Autodesk Fusion 360 part; units mm, degrees
(part 9 of 14)
  arc A2489 (70.5612, 9.5568) -> (70.5612, 10.2553) centre (70.5612, 9.906) ccw
  line L4099 (71.181, 52.94) -> (71.181, 51.54)
  arc A2490 (70.5612, 9.3472) -> (70.5612, 10.4648) centre (70.5612, 9.906) ccw
  line L4100 (83.0072, 9.779) -> (83.5152, 9.779)
  line L4101 (70.3072, 9.906) -> (70.8152, 9.906)
  arc A2491 (70.231, 9.906) -> (70.8914, 9.906) centre (70.5612, 9.906) ccw
  arc A2492 (83.5914, 9.779) -> (82.931, 9.779) centre (83.2612, 9.779) ccw
  line L4102 (70.3072, 9.906) -> (70.8152, 9.906)
  line L4103 (70.5612, 9.652) -> (70.5612, 10.16)
  arc A2493 (70.5612, 10.4648) -> (70.5612, 9.3472) centre (70.5612, 9.906) ccw
  arc A2494 (84.3788, 9.779) -> (82.1436, 9.779) centre (83.2612, 9.779) ccw
  line L4104 (70.5612, 9.652) -> (70.5612, 10.16)
  arc A2495 (71.6788, 9.906) -> (69.4436, 9.906) centre (70.5612, 9.906) ccw
  arc A2496 (83.5914, 9.779) -> (82.931, 9.779) centre (83.2612, 9.779) ccw
  line L4105 (70.3072, 9.906) -> (70.8152, 9.906)
  arc A2497 (70.5612, 10.4648) -> (70.5612, 9.3472) centre (70.5612, 9.906) ccw
  arc A2498 (70.5612, 9.3472) -> (70.5612, 10.4648) centre (70.5612, 9.906) ccw
  arc A2499 (70.231, 9.906) -> (70.8914, 9.906) centre (70.5612, 9.906) ccw
  arc A2500 (70.231, 9.906) -> (70.8914, 9.906) centre (70.5612, 9.906) ccw
  arc A2501 (70.231, 9.906) -> (70.8914, 9.906) centre (70.5612, 9.906) ccw
  line L4106 (71.181, 52.94) -> (71.181, 51.54)
  line L4107 (71.181, 52.94) -> (71.181, 51.54)
  line L4108 (70.5612, 9.652) -> (70.5612, 10.16)
  arc A2502 (72.331, 52.5562) -> (72.331, 51.9238) centre (72.331, 52.24) ccw
  line L4109 (71.181, 55.14) -> (71.181, 53.74)
  arc A2503 (70.5612, 10.4648) -> (70.5612, 9.3472) centre (70.5612, 9.906) ccw
  arc A2504 (70.8914, 9.906) -> (70.231, 9.906) centre (70.5612, 9.906) ccw
  arc A2505 (70.8914, 9.906) -> (70.231, 9.906) centre (70.5612, 9.906) ccw
  line L4110 (71.181, 55.14) -> (71.181, 53.74)
  line L4111 (69.281, 52.94) -> (69.281, 51.54)
  line L4112 (70.3072, 9.906) -> (70.8152, 9.906)
  arc A2506 (70.5612, 10.2553) -> (70.5612, 9.5568) centre (70.5612, 9.906) ccw
  line L4113 (70.3072, 9.906) -> (70.8152, 9.906)
  arc A2507 (70.231, 9.906) -> (70.8914, 9.906) centre (70.5612, 9.906) ccw
  arc A2508 (70.8914, 9.906) -> (70.231, 9.906) centre (70.5612, 9.906) ccw
  line L4114 (69.281, 55.14) -> (69.281, 53.74)
  arc A2509 (83.5914, 9.779) -> (82.931, 9.779) centre (83.2612, 9.779) ccw
  arc A2510 (70.8914, 9.906) -> (70.231, 9.906) centre (70.5612, 9.906) ccw
  line L4115 (70.5612, 9.652) -> (70.5612, 10.16)
  line L4116 (70.3072, 9.906) -> (70.8152, 9.906)
  arc A2511 (82.1436, 9.779) -> (84.3788, 9.779) centre (83.2612, 9.779) ccw
  arc A2512 (82.1436, 9.779) -> (84.3788, 9.779) centre (83.2612, 9.779) ccw
  arc A2513 (82.931, 9.779) -> (83.5914, 9.779) centre (83.2612, 9.779) ccw
  arc A2514 (83.2612, 10.3378) -> (83.2612, 9.2202) centre (83.2612, 9.779) ccw
  arc A2515 (71.6788, 44.45) -> (69.4436, 44.45) centre (70.5612, 44.45) ccw
  arc A2516 (70.8914, 9.906) -> (70.231, 9.906) centre (70.5612, 9.906) ccw
  arc A2517 (82.931, 9.779) -> (83.5914, 9.779) centre (83.2612, 9.779) ccw
  arc A2518 (83.2612, 10.3378) -> (83.2612, 9.2202) centre (83.2612, 9.779) ccw
  arc A2519 (82.931, 9.779) -> (83.5914, 9.779) centre (83.2612, 9.779) ccw
  arc A2520 (83.2612, 9.2202) -> (83.2612, 10.3378) centre (83.2612, 9.779) ccw
  arc A2521 (70.231, 9.906) -> (70.8914, 9.906) centre (70.5612, 9.906) ccw
  arc A2522 (83.2612, 10.3378) -> (83.2612, 9.2202) centre (83.2612, 9.779) ccw
  line L4117 (70.3072, 9.906) -> (70.8152, 9.906)
  line L4118 (70.5612, 9.652) -> (70.5612, 10.16)
  arc A2523 (70.8914, 44.45) -> (70.231, 44.45) centre (70.5612, 44.45) ccw
  line L4119 (70.3072, 44.45) -> (70.8152, 44.45)
  line L4120 (83.0072, 9.779) -> (83.5152, 9.779)
  arc A2524 (83.5914, 9.779) -> (82.931, 9.779) centre (83.2612, 9.779) ccw
  line L4121 (83.2612, 9.525) -> (83.2612, 10.033)
  arc A2525 (83.2612, 9.2202) -> (83.2612, 10.3378) centre (83.2612, 9.779) ccw
  arc A2526 (83.2612, 9.2202) -> (83.2612, 10.3378) centre (83.2612, 9.779) ccw
  arc A2527 (70.8914, 44.45) -> (70.231, 44.45) centre (70.5612, 44.45) ccw
  arc A2528 (70.5612, 9.3472) -> (70.5612, 10.4648) centre (70.5612, 9.906) ccw
  arc A2529 (83.5914, 9.779) -> (82.931, 9.779) centre (83.2612, 9.779) ccw
  arc A2530 (83.2612, 9.2202) -> (83.2612, 10.3378) centre (83.2612, 9.779) ccw
  line L4122 (83.0072, 9.779) -> (83.5152, 9.779)
  arc A2531 (70.231, 44.45) -> (70.8914, 44.45) centre (70.5612, 44.45) ccw
  arc A2532 (82.931, 9.779) -> (83.5914, 9.779) centre (83.2612, 9.779) ccw
  arc A2533 (70.8914, 9.906) -> (70.231, 9.906) centre (70.5612, 9.906) ccw
  arc A2534 (70.231, 44.45) -> (70.8914, 44.45) centre (70.5612, 44.45) ccw
  arc A2535 (69.4436, 44.45) -> (71.6788, 44.45) centre (70.5612, 44.45) ccw
  line L4123 (83.0072, 9.779) -> (83.5152, 9.779)
  arc A2536 (69.4436, 44.45) -> (71.6788, 44.45) centre (70.5612, 44.45) ccw
  arc A2537 (83.5914, 9.779) -> (82.931, 9.779) centre (83.2612, 9.779) ccw
  line L4124 (70.5612, 44.196) -> (70.5612, 44.704)
  line L4125 (83.0072, 9.779) -> (83.5152, 9.779)
  line L4126 (83.2612, 9.525) -> (83.2612, 10.033)
  arc A2538 (71.6788, 44.45) -> (69.4436, 44.45) centre (70.5612, 44.45) ccw
  arc A2539 (71.6788, 44.45) -> (69.4436, 44.45) centre (70.5612, 44.45) ccw
  line L4127 (70.3072, 44.45) -> (70.8152, 44.45)
  arc A2540 (84.3788, 9.779) -> (82.1436, 9.779) centre (83.2612, 9.779) ccw
  line L4128 (83.2612, 9.525) -> (83.2612, 10.033)
  line L4129 (83.0072, 9.779) -> (83.5152, 9.779)
  arc A2541 (70.231, 9.906) -> (70.8914, 9.906) centre (70.5612, 9.906) ccw
  arc A2542 (70.8914, 44.45) -> (70.231, 44.45) centre (70.5612, 44.45) ccw
  arc A2543 (69.4436, 44.45) -> (71.6788, 44.45) centre (70.5612, 44.45) ccw
  line L4130 (83.2612, 9.525) -> (83.2612, 10.033)
  arc A2544 (83.5914, 9.779) -> (82.931, 9.779) centre (83.2612, 9.779) ccw
  arc A2545 (83.2612, 9.2202) -> (83.2612, 10.3378) centre (83.2612, 9.779) ccw
  arc A2546 (82.1436, 9.779) -> (84.3788, 9.779) centre (83.2612, 9.779) ccw
  arc A2547 (82.931, 9.779) -> (83.5914, 9.779) centre (83.2612, 9.779) ccw
  line L4131 (70.3072, 9.906) -> (70.8152, 9.906)
  arc A2548 (70.8914, 44.45) -> (70.231, 44.45) centre (70.5612, 44.45) ccw
  line L4132 (70.5612, 44.196) -> (70.5612, 44.704)
  arc A2549 (70.231, 44.45) -> (70.8914, 44.45) centre (70.5612, 44.45) ccw
  arc A2550 (83.5914, 9.779) -> (82.931, 9.779) centre (83.2612, 9.779) ccw
  arc A2551 (83.2612, 10.1283) -> (83.2612, 9.4298) centre (83.2612, 9.779) ccw
  line L4133 (70.5612, 44.196) -> (70.5612, 44.704)
  arc A2552 (83.5914, 9.779) -> (82.931, 9.779) centre (83.2612, 9.779) ccw
  line L4134 (83.2612, 9.525) -> (83.2612, 10.033)
  arc A2553 (84.3788, 9.779) -> (82.1436, 9.779) centre (83.2612, 9.779) ccw
  line L4135 (70.5612, 9.652) -> (70.5612, 10.16)
  line L4136 (83.2612, 9.525) -> (83.2612, 10.033)
  line L4137 (83.0072, 9.779) -> (83.5152, 9.779)
  line L4138 (83.0072, 9.779) -> (83.5152, 9.779)
  arc A2554 (70.231, 44.45) -> (70.8914, 44.45) centre (70.5612, 44.45) ccw
  arc A2555 (82.931, 44.45) -> (83.5914, 44.45) centre (83.2612, 44.45) ccw
  line L4139 (70.5612, 44.196) -> (70.5612, 44.704)
  line L4140 (83.2612, 44.196) -> (83.2612, 44.704)
  line L4141 (83.0072, 9.779) -> (83.5152, 9.779)
  line L4142 (70.3072, 44.45) -> (70.8152, 44.45)
  arc A2556 (70.231, 44.45) -> (70.8914, 44.45) centre (70.5612, 44.45) ccw
  arc A2557 (82.931, 9.779) -> (83.5914, 9.779) centre (83.2612, 9.779) ccw
  line L4143 (70.5612, 44.196) -> (70.5612, 44.704)
  arc A2558 (70.5612, 43.8912) -> (70.5612, 45.0088) centre (70.5612, 44.45) ccw
  line L4144 (70.3072, 44.45) -> (70.8152, 44.45)
  line L4145 (83.2612, 9.525) -> (83.2612, 10.033)
  line L4146 (70.3072, 44.45) -> (70.8152, 44.45)
  arc A2559 (83.5914, 44.45) -> (82.931, 44.45) centre (83.2612, 44.45) ccw
  arc A2560 (70.8914, 44.45) -> (70.231, 44.45) centre (70.5612, 44.45) ccw
  arc A2561 (83.2612, 9.4298) -> (83.2612, 10.1283) centre (83.2612, 9.779) ccw
  arc A2562 (70.5612, 43.8912) -> (70.5612, 45.0088) centre (70.5612, 44.45) ccw
  arc A2563 (70.231, 44.45) -> (70.8914, 44.45) centre (70.5612, 44.45) ccw
  arc A2564 (70.231, 44.45) -> (70.8914, 44.45) centre (70.5612, 44.45) ccw
  arc A2565 (82.931, 44.45) -> (83.5914, 44.45) centre (83.2612, 44.45) ccw
  arc A2566 (70.8914, 44.45) -> (70.231, 44.45) centre (70.5612, 44.45) ccw
  line L4147 (70.5612, 44.196) -> (70.5612, 44.704)
  arc A2567 (83.2612, 10.3378) -> (83.2612, 9.2202) centre (83.2612, 9.779) ccw
  line L4148 (70.3072, 44.45) -> (70.8152, 44.45)
  arc A2568 (82.931, 44.45) -> (83.5914, 44.45) centre (83.2612, 44.45) ccw
  arc A2569 (70.5612, 43.8912) -> (70.5612, 45.0088) centre (70.5612, 44.45) ccw
  line L4149 (70.3072, 44.45) -> (70.8152, 44.45)
  arc A2570 (82.1436, 44.45) -> (84.3788, 44.45) centre (83.2612, 44.45) ccw
  arc A2571 (84.3788, 44.45) -> (82.1436, 44.45) centre (83.2612, 44.45) ccw
  arc A2572 (70.5612, 45.0088) -> (70.5612, 43.8912) centre (70.5612, 44.45) ccw
  arc A2573 (70.231, 44.45) -> (70.8914, 44.45) centre (70.5612, 44.45) ccw
  arc A2574 (83.5914, 44.45) -> (82.931, 44.45) centre (83.2612, 44.45) ccw
  arc A2575 (70.8914, 44.45) -> (70.231, 44.45) centre (70.5612, 44.45) ccw
  line L4150 (70.5612, 44.196) -> (70.5612, 44.704)
  line L4151 (70.5612, 44.196) -> (70.5612, 44.704)
  arc A2576 (70.5612, 44.7993) -> (70.5612, 44.1007) centre (70.5612, 44.45) ccw
  arc A2577 (70.8914, 44.45) -> (70.231, 44.45) centre (70.5612, 44.45) ccw
  arc A2578 (70.5612, 45.0088) -> (70.5612, 43.8912) centre (70.5612, 44.45) ccw
  arc A2579 (82.931, 44.45) -> (83.5914, 44.45) centre (83.2612, 44.45) ccw
  arc A2580 (70.5612, 44.1007) -> (70.5612, 44.7993) centre (70.5612, 44.45) ccw
  line L4152 (70.5612, 44.196) -> (70.5612, 44.704)
  line L4153 (70.3072, 44.45) -> (70.8152, 44.45)
  arc A2581 (83.5914, 9.779) -> (82.931, 9.779) centre (83.2612, 9.779) ccw
  arc A2582 (84.3788, 44.45) -> (82.1436, 44.45) centre (83.2612, 44.45) ccw
  arc A2583 (70.5612, 43.8912) -> (70.5612, 45.0088) centre (70.5612, 44.45) ccw
  arc A2584 (70.5612, 45.0088) -> (70.5612, 43.8912) centre (70.5612, 44.45) ccw
  line L4154 (83.0072, 44.45) -> (83.5152, 44.45)
  arc A2585 (70.231, 44.45) -> (70.8914, 44.45) centre (70.5612, 44.45) ccw
  arc A2586 (70.5612, 45.0088) -> (70.5612, 43.8912) centre (70.5612, 44.45) ccw
  arc A2587 (70.8914, 44.45) -> (70.231, 44.45) centre (70.5612, 44.45) ccw
  line L4155 (70.5612, 44.196) -> (70.5612, 44.704)
  line L4156 (83.2612, 44.196) -> (83.2612, 44.704)
  arc A2588 (82.1436, 44.45) -> (84.3788, 44.45) centre (83.2612, 44.45) ccw
  line L4157 (70.3072, 44.45) -> (70.8152, 44.45)
  arc A2589 (70.5612, 45.0088) -> (70.5612, 43.8912) centre (70.5612, 44.45) ccw
  arc A2590 (70.8914, 44.45) -> (70.231, 44.45) centre (70.5612, 44.45) ccw
  arc A2591 (70.5612, 43.8912) -> (70.5612, 45.0088) centre (70.5612, 44.45) ccw
  arc A2592 (84.3788, 44.45) -> (82.1436, 44.45) centre (83.2612, 44.45) ccw
  line L4158 (70.3072, 44.45) -> (70.8152, 44.45)
  arc A2593 (82.1436, 44.45) -> (84.3788, 44.45) centre (83.2612, 44.45) ccw
  arc A2594 (83.2612, 10.3378) -> (83.2612, 9.2202) centre (83.2612, 9.779) ccw
  line L4159 (83.0072, 44.45) -> (83.5152, 44.45)
  arc A2595 (70.231, 44.45) -> (70.8914, 44.45) centre (70.5612, 44.45) ccw
  arc A2596 (83.5914, 44.45) -> (82.931, 44.45) centre (83.2612, 44.45) ccw
  line L4160 (83.0072, 44.45) -> (83.5152, 44.45)
  arc A2597 (83.2612, 43.8912) -> (83.2612, 45.0088) centre (83.2612, 44.45) ccw
  arc A2598 (67.0306, 27.1272) -> (64.7954, 27.1272) centre (65.913, 27.1272) ccw
  line L4161 (83.2612, 44.196) -> (83.2612, 44.704)
  arc A2599 (82.931, 44.45) -> (83.5914, 44.45) centre (83.2612, 44.45) ccw
  line L4162 (83.0072, 44.45) -> (83.5152, 44.45)
  arc A2600 (66.2432, 27.1272) -> (65.5828, 27.1272) centre (65.913, 27.1272) ccw
  arc A2601 (83.5914, 44.45) -> (82.931, 44.45) centre (83.2612, 44.45) ccw
  arc A2602 (65.5828, 27.1272) -> (66.2432, 27.1272) centre (65.913, 27.1272) ccw
  arc A2603 (64.7954, 14.4272) -> (67.0306, 14.4272) centre (65.913, 14.4272) ccw
  arc A2604 (65.5828, 14.4272) -> (66.2432, 14.4272) centre (65.913, 14.4272) ccw
  arc A2605 (83.2612, 43.8912) -> (83.2612, 45.0088) centre (83.2612, 44.45) ccw
  arc A2606 (82.931, 44.45) -> (83.5914, 44.45) centre (83.2612, 44.45) ccw
  line L4163 (83.0072, 44.45) -> (83.5152, 44.45)
  arc A2607 (83.5914, 44.45) -> (82.931, 44.45) centre (83.2612, 44.45) ccw
  arc A2608 (82.931, 44.45) -> (83.5914, 44.45) centre (83.2612, 44.45) ccw
  arc A2609 (83.2612, 45.0088) -> (83.2612, 43.8912) centre (83.2612, 44.45) ccw
  arc A2610 (67.0306, 27.1272) -> (64.7954, 27.1272) centre (65.913, 27.1272) ccw
  line L4164 (83.2612, 44.196) -> (83.2612, 44.704)
  arc A2611 (67.0306, 27.1272) -> (64.7954, 27.1272) centre (65.913, 27.1272) ccw
  arc A2612 (83.5914, 44.45) -> (82.931, 44.45) centre (83.2612, 44.45) ccw
  arc A2613 (66.2432, 27.1272) -> (65.5828, 27.1272) centre (65.913, 27.1272) ccw
  line L4165 (83.0072, 44.45) -> (83.5152, 44.45)
  arc A2614 (65.5828, 27.1272) -> (66.2432, 27.1272) centre (65.913, 27.1272) ccw
  line L4166 (65.659, 27.1272) -> (66.167, 27.1272)
  arc A2615 (83.2612, 44.1007) -> (83.2612, 44.7993) centre (83.2612, 44.45) ccw
  arc A2616 (83.5914, 44.45) -> (82.931, 44.45) centre (83.2612, 44.45) ccw
  line L4167 (65.913, 26.8732) -> (65.913, 27.3812)
  arc A2617 (66.2432, 27.1272) -> (65.5828, 27.1272) centre (65.913, 27.1272) ccw
  arc A2618 (65.5828, 14.4272) -> (66.2432, 14.4272) centre (65.913, 14.4272) ccw
  arc A2619 (82.931, 44.45) -> (83.5914, 44.45) centre (83.2612, 44.45) ccw
  line L4168 (65.913, 26.8732) -> (65.913, 27.3812)
  arc A2620 (83.2612, 43.8912) -> (83.2612, 45.0088) centre (83.2612, 44.45) ccw
  line L4169 (83.0072, 44.45) -> (83.5152, 44.45)
  arc A2621 (64.7954, 27.1272) -> (67.0306, 27.1272) centre (65.913, 27.1272) ccw
  arc A2622 (66.2432, 27.1272) -> (65.5828, 27.1272) centre (65.913, 27.1272) ccw
  line L4170 (83.0072, 44.45) -> (83.5152, 44.45)
  line L4171 (65.913, 26.8732) -> (65.913, 27.3812)
  arc A2623 (83.5914, 44.45) -> (82.931, 44.45) centre (83.2612, 44.45) ccw
  line L4172 (83.0072, 44.45) -> (83.5152, 44.45)
  arc A2624 (83.2612, 45.0088) -> (83.2612, 43.8912) centre (83.2612, 44.45) ccw
  arc A2625 (64.7954, 27.1272) -> (67.0306, 27.1272) centre (65.913, 27.1272) ccw
  line L4173 (83.2612, 44.196) -> (83.2612, 44.704)
  arc A2626 (64.7954, 27.1272) -> (67.0306, 27.1272) centre (65.913, 27.1272) ccw
  arc A2627 (66.2432, 27.1272) -> (65.5828, 27.1272) centre (65.913, 27.1272) ccw
  arc A2628 (83.5914, 44.45) -> (82.931, 44.45) centre (83.2612, 44.45) ccw
  line L4174 (65.913, 26.8732) -> (65.913, 27.3812)
  line L4175 (83.2612, 44.196) -> (83.2612, 44.704)
  arc A2629 (83.2612, 43.8912) -> (83.2612, 45.0088) centre (83.2612, 44.45) ccw
  line L4176 (83.0072, 44.45) -> (83.5152, 44.45)
  arc A2630 (83.2612, 45.0088) -> (83.2612, 43.8912) centre (83.2612, 44.45) ccw
  arc A2631 (83.2612, 45.0088) -> (83.2612, 43.8912) centre (83.2612, 44.45) ccw
  line L4177 (83.2612, 44.196) -> (83.2612, 44.704)
  arc A2632 (82.931, 44.45) -> (83.5914, 44.45) centre (83.2612, 44.45) ccw
  arc A2633 (83.2612, 43.8912) -> (83.2612, 45.0088) centre (83.2612, 44.45) ccw
  line L4178 (83.2612, 44.196) -> (83.2612, 44.704)
  arc A2634 (83.2612, 45.0088) -> (83.2612, 43.8912) centre (83.2612, 44.45) ccw
  arc A2635 (83.2612, 44.7993) -> (83.2612, 44.1007) centre (83.2612, 44.45) ccw
  line L4179 (83.2612, 44.196) -> (83.2612, 44.704)
  arc A2636 (82.931, 44.45) -> (83.5914, 44.45) centre (83.2612, 44.45) ccw
  arc A2637 (83.5914, 44.45) -> (82.931, 44.45) centre (83.2612, 44.45) ccw
  line L4180 (65.913, 26.8732) -> (65.913, 27.3812)
  arc A2638 (65.5828, 27.1272) -> (66.2432, 27.1272) centre (65.913, 27.1272) ccw
  line L4181 (83.2612, 44.196) -> (83.2612, 44.704)
  line L4182 (65.659, 27.1272) -> (66.167, 27.1272)
  arc A2639 (64.7954, 39.8272) -> (67.0306, 39.8272) centre (65.913, 39.8272) ccw
  arc A2640 (65.5828, 14.4272) -> (66.2432, 14.4272) centre (65.913, 14.4272) ccw
  arc A2641 (64.7954, 39.8272) -> (67.0306, 39.8272) centre (65.913, 39.8272) ccw
  arc A2642 (65.913, 26.5684) -> (65.913, 27.686) centre (65.913, 27.1272) ccw
  line L4183 (65.659, 14.4272) -> (66.167, 14.4272)
  line L4184 (65.913, 14.1732) -> (65.913, 14.6812)
  arc A2643 (66.2432, 27.1272) -> (65.5828, 27.1272) centre (65.913, 27.1272) ccw
  arc A2644 (66.2432, 27.1272) -> (65.5828, 27.1272) centre (65.913, 27.1272) ccw
  arc A2645 (65.5828, 14.4272) -> (66.2432, 14.4272) centre (65.913, 14.4272) ccw
  arc A2646 (66.2432, 14.4272) -> (65.5828, 14.4272) centre (65.913, 14.4272) ccw
  arc A2647 (65.913, 27.4764) -> (65.913, 26.7779) centre (65.913, 27.1272) ccw
  arc A2648 (65.5828, 27.1272) -> (66.2432, 27.1272) centre (65.913, 27.1272) ccw
  arc A2649 (67.0306, 14.4272) -> (64.7954, 14.4272) centre (65.913, 14.4272) ccw
  line L4185 (65.659, 27.1272) -> (66.167, 27.1272)
  line L4186 (65.659, 27.1272) -> (66.167, 27.1272)
  arc A2650 (66.2432, 27.1272) -> (65.5828, 27.1272) centre (65.913, 27.1272) ccw
  arc A2651 (65.5828, 27.1272) -> (66.2432, 27.1272) centre (65.913, 27.1272) ccw
  line L4187 (65.913, 26.8732) -> (65.913, 27.3812)
  arc A2652 (65.5828, 14.4272) -> (66.2432, 14.4272) centre (65.913, 14.4272) ccw
  arc A2653 (65.913, 26.5684) -> (65.913, 27.686) centre (65.913, 27.1272) ccw
  arc A2654 (65.913, 27.686) -> (65.913, 26.5684) centre (65.913, 27.1272) ccw
  arc A2655 (65.5828, 27.1272) -> (66.2432, 27.1272) centre (65.913, 27.1272) ccw
  arc A2656 (66.2432, 27.1272) -> (65.5828, 27.1272) centre (65.913, 27.1272) ccw
  arc A2657 (66.2432, 14.4272) -> (65.5828, 14.4272) centre (65.913, 14.4272) ccw
  line L4188 (65.913, 14.1732) -> (65.913, 14.6812)
  arc A2658 (66.2432, 14.4272) -> (65.5828, 14.4272) centre (65.913, 14.4272) ccw
  arc A2659 (66.2432, 14.4272) -> (65.5828, 14.4272) centre (65.913, 14.4272) ccw
  line L4189 (65.659, 14.4272) -> (66.167, 14.4272)
  line L4190 (65.659, 14.4272) -> (66.167, 14.4272)
  arc A2660 (65.5828, 27.1272) -> (66.2432, 27.1272) centre (65.913, 27.1272) ccw
  line L4191 (65.913, 14.1732) -> (65.913, 14.6812)
  arc A2661 (65.913, 26.7779) -> (65.913, 27.4764) centre (65.913, 27.1272) ccw
  line L4192 (65.659, 27.1272) -> (66.167, 27.1272)
  arc A2662 (65.913, 27.686) -> (65.913, 26.5684) centre (65.913, 27.1272) ccw
  arc A2663 (65.913, 26.5684) -> (65.913, 27.686) centre (65.913, 27.1272) ccw
  arc A2664 (65.5828, 14.4272) -> (66.2432, 14.4272) centre (65.913, 14.4272) ccw
  line L4193 (65.659, 14.4272) -> (66.167, 14.4272)
  line L4194 (65.659, 27.1272) -> (66.167, 27.1272)
  arc A2665 (64.7954, 14.4272) -> (67.0306, 14.4272) centre (65.913, 14.4272) ccw
  arc A2666 (65.913, 27.686) -> (65.913, 26.5684) centre (65.913, 27.1272) ccw
  line L4195 (65.913, 26.8732) -> (65.913, 27.3812)
  line L4196 (65.659, 27.1272) -> (66.167, 27.1272)
  arc A2667 (65.5828, 14.4272) -> (66.2432, 14.4272) centre (65.913, 14.4272) ccw
  line L4197 (65.659, 14.4272) -> (66.167, 14.4272)
  line L4198 (65.659, 27.1272) -> (66.167, 27.1272)
  line L4199 (65.659, 14.4272) -> (66.167, 14.4272)
  arc A2668 (64.7954, 14.4272) -> (67.0306, 14.4272) centre (65.913, 14.4272) ccw
  arc A2669 (65.913, 27.686) -> (65.913, 26.5684) centre (65.913, 27.1272) ccw
  line L4200 (65.913, 26.8732) -> (65.913, 27.3812)
  arc A2670 (67.0306, 14.4272) -> (64.7954, 14.4272) centre (65.913, 14.4272) ccw
  arc A2671 (67.0306, 14.4272) -> (64.7954, 14.4272) centre (65.913, 14.4272) ccw
  line L4201 (65.659, 27.1272) -> (66.167, 27.1272)
  arc A2672 (66.2432, 27.1272) -> (65.5828, 27.1272) centre (65.913, 27.1272) ccw
  line L4202 (65.913, 26.8732) -> (65.913, 27.3812)
  arc A2673 (65.913, 26.5684) -> (65.913, 27.686) centre (65.913, 27.1272) ccw
  line L4203 (65.913, 14.1732) -> (65.913, 14.6812)
  arc A2674 (65.5828, 27.1272) -> (66.2432, 27.1272) centre (65.913, 27.1272) ccw
  line L4204 (65.659, 27.1272) -> (66.167, 27.1272)
  arc A2675 (65.913, 26.5684) -> (65.913, 27.686) centre (65.913, 27.1272) ccw
  arc A2676 (65.5828, 27.1272) -> (66.2432, 27.1272) centre (65.913, 27.1272) ccw
  arc A2677 (66.2432, 14.4272) -> (65.5828, 14.4272) centre (65.913, 14.4272) ccw
  arc A2678 (65.5828, 27.1272) -> (66.2432, 27.1272) centre (65.913, 27.1272) ccw
  arc A2679 (65.913, 27.686) -> (65.913, 26.5684) centre (65.913, 27.1272) ccw
  line L4205 (65.913, 26.8732) -> (65.913, 27.3812)
  line L4206 (65.913, 39.5732) -> (65.913, 40.0812)
  arc A2680 (66.2432, 39.8272) -> (65.5828, 39.8272) centre (65.913, 39.8272) ccw
  line L4207 (65.913, 39.5732) -> (65.913, 40.0812)
  arc A2681 (65.5828, 39.8272) -> (66.2432, 39.8272) centre (65.913, 39.8272) ccw
  line L4208 (65.659, 39.8272) -> (66.167, 39.8272)
  arc A2682 (65.913, 13.8684) -> (65.913, 14.986) centre (65.913, 14.4272) ccw
  arc A2683 (64.7954, 39.8272) -> (67.0306, 39.8272) centre (65.913, 39.8272) ccw
  arc A2684 (65.913, 14.986) -> (65.913, 13.8684) centre (65.913, 14.4272) ccw
  line L4209 (65.913, 14.1732) -> (65.913, 14.6812)
  arc A2685 (65.913, 14.986) -> (65.913, 13.8684) centre (65.913, 14.4272) ccw
  arc A2686 (65.5828, 14.4272) -> (66.2432, 14.4272) centre (65.913, 14.4272) ccw
  arc A2687 (66.2432, 39.8272) -> (65.5828, 39.8272) centre (65.913, 39.8272) ccw
  arc A2688 (65.5828, 39.8272) -> (66.2432, 39.8272) centre (65.913, 39.8272) ccw
  line L4210 (65.659, 39.8272) -> (66.167, 39.8272)
  arc A2689 (66.2432, 14.4272) -> (65.5828, 14.4272) centre (65.913, 14.4272) ccw
  arc A2690 (65.5828, 14.4272) -> (66.2432, 14.4272) centre (65.913, 14.4272) ccw
  line L4211 (65.659, 39.8272) -> (66.167, 39.8272)
  arc A2691 (66.2432, 39.8272) -> (65.5828, 39.8272) centre (65.913, 39.8272) ccw
  line L4212 (65.913, 14.1732) -> (65.913, 14.6812)
  line L4213 (65.659, 39.8272) -> (66.167, 39.8272)
  arc A2692 (65.913, 40.386) -> (65.913, 39.2684) centre (65.913, 39.8272) ccw
  arc A2693 (65.913, 13.8684) -> (65.913, 14.986) centre (65.913, 14.4272) ccw
  arc A2694 (65.5828, 39.8272) -> (66.2432, 39.8272) centre (65.913, 39.8272) ccw
  arc A2695 (65.913, 40.386) -> (65.913, 39.2684) centre (65.913, 39.8272) ccw
  arc A2696 (65.913, 39.2684) -> (65.913, 40.386) centre (65.913, 39.8272) ccw
  arc A2697 (66.2432, 39.8272) -> (65.5828, 39.8272) centre (65.913, 39.8272) ccw
  arc A2698 (66.2432, 39.8272) -> (65.5828, 39.8272) centre (65.913, 39.8272) ccw
  line L4214 (65.913, 39.5732) -> (65.913, 40.0812)
  line L4215 (65.913, 14.1732) -> (65.913, 14.6812)
  arc A2699 (65.913, 14.986) -> (65.913, 13.8684) centre (65.913, 14.4272) ccw
  arc A2700 (65.913, 39.478) -> (65.913, 40.1765) centre (65.913, 39.8272) ccw
  arc A2701 (65.5828, 39.8272) -> (66.2432, 39.8272) centre (65.913, 39.8272) ccw
  arc A2702 (65.913, 40.386) -> (65.913, 39.2684) centre (65.913, 39.8272) ccw
  arc A2703 (66.2432, 39.8272) -> (65.5828, 39.8272) centre (65.913, 39.8272) ccw
  line L4216 (65.659, 39.8272) -> (66.167, 39.8272)
  line L4217 (65.913, 14.1732) -> (65.913, 14.6812)
  arc A2704 (65.913, 13.8684) -> (65.913, 14.986) centre (65.913, 14.4272) ccw
  line L4218 (65.659, 14.4272) -> (66.167, 14.4272)
  arc A2705 (67.0306, 39.8272) -> (64.7954, 39.8272) centre (65.913, 39.8272) ccw
  arc A2706 (65.913, 13.8684) -> (65.913, 14.986) centre (65.913, 14.4272) ccw
  arc A2707 (65.913, 14.7765) -> (65.913, 14.0779) centre (65.913, 14.4272) ccw
  arc A2708 (66.2432, 14.4272) -> (65.5828, 14.4272) centre (65.913, 14.4272) ccw
  arc A2709 (65.913, 14.986) -> (65.913, 13.8684) centre (65.913, 14.4272) ccw
  line L4219 (65.913, 14.1732) -> (65.913, 14.6812)
  arc A2710 (65.913, 14.986) -> (65.913, 13.8684) centre (65.913, 14.4272) ccw
  arc A2711 (65.913, 13.8684) -> (65.913, 14.986) centre (65.913, 14.4272) ccw
  arc A2712 (65.5828, 39.8272) -> (66.2432, 39.8272) centre (65.913, 39.8272) ccw
  arc A2713 (66.2432, 14.4272) -> (65.5828, 14.4272) centre (65.913, 14.4272) ccw
  arc A2714 (66.2432, 39.8272) -> (65.5828, 39.8272) centre (65.913, 39.8272) ccw
  line L4220 (65.659, 14.4272) -> (66.167, 14.4272)
  line L4221 (65.913, 14.1732) -> (65.913, 14.6812)
  arc A2715 (65.913, 14.0779) -> (65.913, 14.7765) centre (65.913, 14.4272) ccw
  line L4222 (65.913, 39.5732) -> (65.913, 40.0812)
  arc A2716 (67.0306, 39.8272) -> (64.7954, 39.8272) centre (65.913, 39.8272) ccw
  line L4223 (65.659, 14.4272) -> (66.167, 14.4272)
  line L4224 (65.659, 14.4272) -> (66.167, 14.4272)
  arc A2717 (66.2432, 14.4272) -> (65.5828, 14.4272) centre (65.913, 14.4272) ccw
  arc A2718 (66.2432, 14.4272) -> (65.5828, 14.4272) centre (65.913, 14.4272) ccw
  line L4225 (65.913, 39.5732) -> (65.913, 40.0812)
  arc A2719 (65.5828, 39.8272) -> (66.2432, 39.8272) centre (65.913, 39.8272) ccw
  arc A2720 (65.5828, 14.4272) -> (66.2432, 14.4272) centre (65.913, 14.4272) ccw
  arc A2721 (66.2432, 39.8272) -> (65.5828, 39.8272) centre (65.913, 39.8272) ccw
  arc A2722 (67.0306, 39.8272) -> (64.7954, 39.8272) centre (65.913, 39.8272) ccw
  line L4226 (65.913, 39.5732) -> (65.913, 40.0812)
  line L4227 (87.63, 39.8272) -> (88.138, 39.8272)
  arc A2723 (88.2142, 39.8272) -> (87.5538, 39.8272) centre (87.884, 39.8272) ccw
  arc A2724 (86.7664, 39.8272) -> (89.0016, 39.8272) centre (87.884, 39.8272) ccw
  arc A2725 (87.5538, 39.8272) -> (88.2142, 39.8272) centre (87.884, 39.8272) ccw
  line L4228 (65.913, 39.5732) -> (65.913, 40.0812)
  arc A2726 (87.5538, 39.8272) -> (88.2142, 39.8272) centre (87.884, 39.8272) ccw
  line L4229 (87.63, 39.8272) -> (88.138, 39.8272)
  arc A2727 (89.0016, 39.8272) -> (86.7664, 39.8272) centre (87.884, 39.8272) ccw
  line L4230 (87.884, 39.5732) -> (87.884, 40.0812)
  arc A2728 (87.884, 40.386) -> (87.884, 39.2684) centre (87.884, 39.8272) ccw
  arc A2729 (87.5538, 39.8272) -> (88.2142, 39.8272) centre (87.884, 39.8272) ccw
  arc A2730 (86.7664, 39.8272) -> (89.0016, 39.8272) centre (87.884, 39.8272) ccw
  line L4231 (65.659, 39.8272) -> (66.167, 39.8272)
  arc A2731 (65.913, 39.2684) -> (65.913, 40.386) centre (65.913, 39.8272) ccw
  arc A2732 (65.913, 40.1765) -> (65.913, 39.478) centre (65.913, 39.8272) ccw
  arc A2733 (88.2142, 39.8272) -> (87.5538, 39.8272) centre (87.884, 39.8272) ccw
  arc A2734 (65.913, 39.2684) -> (65.913, 40.386) centre (65.913, 39.8272) ccw
  arc A2735 (87.884, 39.478) -> (87.884, 40.1765) centre (87.884, 39.8272) ccw
  arc A2736 (87.884, 39.2684) -> (87.884, 40.386) centre (87.884, 39.8272) ccw
  line L4232 (87.884, 39.5732) -> (87.884, 40.0812)
  line L4233 (65.659, 39.8272) -> (66.167, 39.8272)
  arc A2737 (87.5538, 39.8272) -> (88.2142, 39.8272) centre (87.884, 39.8272) ccw
  arc A2738 (86.7664, 27.1272) -> (89.0016, 27.1272) centre (87.884, 27.1272) ccw
  line L4234 (87.884, 39.5732) -> (87.884, 40.0812)
  line L4235 (87.884, 39.5732) -> (87.884, 40.0812)
  arc A2739 (87.884, 39.2684) -> (87.884, 40.386) centre (87.884, 39.8272) ccw
  arc A2740 (87.5538, 39.8272) -> (88.2142, 39.8272) centre (87.884, 39.8272) ccw
  arc A2741 (88.2142, 39.8272) -> (87.5538, 39.8272) centre (87.884, 39.8272) ccw
  line L4236 (87.63, 39.8272) -> (88.138, 39.8272)
  line L4237 (65.913, 39.5732) -> (65.913, 40.0812)
  arc A2742 (89.0016, 39.8272) -> (86.7664, 39.8272) centre (87.884, 39.8272) ccw
  arc A2743 (65.5828, 39.8272) -> (66.2432, 39.8272) centre (65.913, 39.8272) ccw
  line L4238 (65.913, 39.5732) -> (65.913, 40.0812)
  arc A2744 (65.913, 39.2684) -> (65.913, 40.386) centre (65.913, 39.8272) ccw
  line L4239 (65.659, 39.8272) -> (66.167, 39.8272)
  arc A2745 (65.5828, 39.8272) -> (66.2432, 39.8272) centre (65.913, 39.8272) ccw
  arc A2746 (65.913, 40.386) -> (65.913, 39.2684) centre (65.913, 39.8272) ccw
  arc A2747 (66.2432, 39.8272) -> (65.5828, 39.8272) centre (65.913, 39.8272) ccw
  arc A2748 (86.7664, 27.1272) -> (89.0016, 27.1272) centre (87.884, 27.1272) ccw
  arc A2749 (87.5538, 39.8272) -> (88.2142, 39.8272) centre (87.884, 39.8272) ccw
  arc A2750 (87.884, 40.386) -> (87.884, 39.2684) centre (87.884, 39.8272) ccw
  arc A2751 (87.884, 39.2684) -> (87.884, 40.386) centre (87.884, 39.8272) ccw
  line L4240 (65.913, 39.5732) -> (65.913, 40.0812)
  arc A2752 (86.7664, 39.8272) -> (89.0016, 39.8272) centre (87.884, 39.8272) ccw
  line L4241 (87.884, 39.5732) -> (87.884, 40.0812)
  arc A2753 (88.2142, 39.8272) -> (87.5538, 39.8272) centre (87.884, 39.8272) ccw
  arc A2754 (87.5538, 39.8272) -> (88.2142, 39.8272) centre (87.884, 39.8272) ccw
  line L4242 (87.63, 39.8272) -> (88.138, 39.8272)
  arc A2755 (87.884, 40.1765) -> (87.884, 39.478) centre (87.884, 39.8272) ccw
  arc A2756 (65.5828, 39.8272) -> (66.2432, 39.8272) centre (65.913, 39.8272) ccw
  arc A2757 (89.0016, 39.8272) -> (86.7664, 39.8272) centre (87.884, 39.8272) ccw
  line L4243 (65.659, 39.8272) -> (66.167, 39.8272)
  arc A2758 (87.884, 39.2684) -> (87.884, 40.386) centre (87.884, 39.8272) ccw
  line L4244 (87.63, 39.8272) -> (88.138, 39.8272)
  arc A2759 (66.2432, 39.8272) -> (65.5828, 39.8272) centre (65.913, 39.8272) ccw
  line L4245 (65.659, 39.8272) -> (66.167, 39.8272)
  arc A2760 (89.0016, 27.1272) -> (86.7664, 27.1272) centre (87.884, 27.1272) ccw
  arc A2761 (65.5828, 39.8272) -> (66.2432, 39.8272) centre (65.913, 39.8272) ccw
  arc A2762 (65.913, 40.386) -> (65.913, 39.2684) centre (65.913, 39.8272) ccw
  arc A2763 (65.913, 39.2684) -> (65.913, 40.386) centre (65.913, 39.8272) ccw
  arc A2764 (87.5538, 39.8272) -> (88.2142, 39.8272) centre (87.884, 39.8272) ccw
  arc A2765 (87.884, 40.386) -> (87.884, 39.2684) centre (87.884, 39.8272) ccw
  arc A2766 (87.884, 40.386) -> (87.884, 39.2684) centre (87.884, 39.8272) ccw
  arc A2767 (87.884, 39.2684) -> (87.884, 40.386) centre (87.884, 39.8272) ccw
  arc A2768 (87.884, 26.7779) -> (87.884, 27.4764) centre (87.884, 27.1272) ccw
  arc A2769 (88.2142, 39.8272) -> (87.5538, 39.8272) centre (87.884, 39.8272) ccw
  arc A2770 (87.884, 27.4764) -> (87.884, 26.7779) centre (87.884, 27.1272) ccw
  arc A2771 (87.5538, 39.8272) -> (88.2142, 39.8272) centre (87.884, 39.8272) ccw
  line L4246 (87.884, 39.5732) -> (87.884, 40.0812)
  line L4247 (87.63, 39.8272) -> (88.138, 39.8272)
  arc A2772 (88.2142, 39.8272) -> (87.5538, 39.8272) centre (87.884, 39.8272) ccw
  arc A2773 (87.884, 27.686) -> (87.884, 26.5684) centre (87.884, 27.1272) ccw
  arc A2774 (86.7664, 14.4272) -> (89.0016, 14.4272) centre (87.884, 14.4272) ccw
  line L4248 (87.63, 27.1272) -> (88.138, 27.1272)
  arc A2775 (88.2142, 27.1272) -> (87.5538, 27.1272) centre (87.884, 27.1272) ccw
  line L4249 (87.63, 27.1272) -> (88.138, 27.1272)
  arc A2776 (88.2142, 27.1272) -> (87.5538, 27.1272) centre (87.884, 27.1272) ccw
  line L4250 (87.63, 27.1272) -> (88.138, 27.1272)
  line L4251 (87.63, 39.8272) -> (88.138, 39.8272)
  arc A2777 (87.5538, 27.1272) -> (88.2142, 27.1272) centre (87.884, 27.1272) ccw
  arc A2778 (86.7664, 27.1272) -> (89.0016, 27.1272) centre (87.884, 27.1272) ccw
  arc A2779 (88.2142, 27.1272) -> (87.5538, 27.1272) centre (87.884, 27.1272) ccw
  arc A2780 (87.884, 26.5684) -> (87.884, 27.686) centre (87.884, 27.1272) ccw
  arc A2781 (89.0016, 14.4272) -> (86.7664, 14.4272) centre (87.884, 14.4272) ccw
  line L4252 (87.884, 39.5732) -> (87.884, 40.0812)
  line L4253 (87.63, 27.1272) -> (88.138, 27.1272)
  line L4254 (87.884, 26.8732) -> (87.884, 27.3812)
  line L4255 (87.884, 26.8732) -> (87.884, 27.3812)
  arc A2782 (88.2142, 27.1272) -> (87.5538, 27.1272) centre (87.884, 27.1272) ccw
  arc A2783 (87.5538, 27.1272) -> (88.2142, 27.1272) centre (87.884, 27.1272) ccw
  arc A2784 (88.2142, 27.1272) -> (87.5538, 27.1272) centre (87.884, 27.1272) ccw
  line L4256 (87.884, 26.8732) -> (87.884, 27.3812)
  arc A2785 (87.884, 26.5684) -> (87.884, 27.686) centre (87.884, 27.1272) ccw
  line L4257 (87.63, 39.8272) -> (88.138, 39.8272)
  arc A2786 (87.5538, 27.1272) -> (88.2142, 27.1272) centre (87.884, 27.1272) ccw
  line L4258 (87.63, 27.1272) -> (88.138, 27.1272)
  line L4259 (87.884, 26.8732) -> (87.884, 27.3812)
  arc A2787 (87.5538, 27.1272) -> (88.2142, 27.1272) centre (87.884, 27.1272) ccw
  arc A2788 (88.2142, 39.8272) -> (87.5538, 39.8272) centre (87.884, 39.8272) ccw
  arc A2789 (87.884, 27.686) -> (87.884, 26.5684) centre (87.884, 27.1272) ccw
  line L4260 (87.884, 26.8732) -> (87.884, 27.3812)
  arc A2790 (89.0016, 27.1272) -> (86.7664, 27.1272) centre (87.884, 27.1272) ccw
  line L4261 (87.63, 39.8272) -> (88.138, 39.8272)
  line L4262 (87.63, 39.8272) -> (88.138, 39.8272)
  arc A2791 (87.5538, 39.8272) -> (88.2142, 39.8272) centre (87.884, 39.8272) ccw
  arc A2792 (87.5538, 27.1272) -> (88.2142, 27.1272) centre (87.884, 27.1272) ccw
  arc A2793 (87.5538, 27.1272) -> (88.2142, 27.1272) centre (87.884, 27.1272) ccw
  line L4263 (87.63, 27.1272) -> (88.138, 27.1272)
  line L4264 (87.884, 39.5732) -> (87.884, 40.0812)
  arc A2794 (88.2142, 27.1272) -> (87.5538, 27.1272) centre (87.884, 27.1272) ccw
  arc A2795 (87.884, 40.386) -> (87.884, 39.2684) centre (87.884, 39.8272) ccw
  arc A2796 (88.2142, 39.8272) -> (87.5538, 39.8272) centre (87.884, 39.8272) ccw
  line L4265 (87.63, 27.1272) -> (88.138, 27.1272)
  arc A2797 (87.5538, 27.1272) -> (88.2142, 27.1272) centre (87.884, 27.1272) ccw
  arc A2798 (88.2142, 27.1272) -> (87.5538, 27.1272) centre (87.884, 27.1272) ccw
  arc A2799 (89.0016, 27.1272) -> (86.7664, 27.1272) centre (87.884, 27.1272) ccw
  arc A2800 (88.2142, 39.8272) -> (87.5538, 39.8272) centre (87.884, 39.8272) ccw
  line L4266 (87.884, 39.5732) -> (87.884, 40.0812)
  line L4267 (87.884, 26.8732) -> (87.884, 27.3812)
  arc A2801 (88.2142, 27.1272) -> (87.5538, 27.1272) centre (87.884, 27.1272) ccw
  line L4268 (87.884, 26.8732) -> (87.884, 27.3812)
  line L4269 (87.884, 39.5732) -> (87.884, 40.0812)
  arc A2802 (87.5538, 27.1272) -> (88.2142, 27.1272) centre (87.884, 27.1272) ccw
  line L4270 (87.63, 27.1272) -> (88.138, 27.1272)
  arc A2803 (88.2142, 27.1272) -> (87.5538, 27.1272) centre (87.884, 27.1272) ccw
  arc A2804 (87.5538, 27.1272) -> (88.2142, 27.1272) centre (87.884, 27.1272) ccw
  arc A2805 (88.2142, 39.8272) -> (87.5538, 39.8272) centre (87.884, 39.8272) ccw
  line L4271 (87.884, 26.8732) -> (87.884, 27.3812)
  line L4272 (87.884, 14.1732) -> (87.884, 14.6812)
  line L4273 (87.884, 14.1732) -> (87.884, 14.6812)
  arc A2806 (88.2142, 14.4272) -> (87.5538, 14.4272) centre (87.884, 14.4272) ccw
  arc A2807 (88.2142, 14.4272) -> (87.5538, 14.4272) centre (87.884, 14.4272) ccw
  line L4274 (87.884, 14.1732) -> (87.884, 14.6812)
  arc A2808 (87.5538, 14.4272) -> (88.2142, 14.4272) centre (87.884, 14.4272) ccw
  line L4275 (87.63, 14.4272) -> (88.138, 14.4272)
  arc A2809 (87.884, 27.686) -> (87.884, 26.5684) centre (87.884, 27.1272) ccw
  arc A2810 (89.0016, 14.4272) -> (86.7664, 14.4272) centre (87.884, 14.4272) ccw
  arc A2811 (88.2142, 14.4272) -> (87.5538, 14.4272) centre (87.884, 14.4272) ccw
  line L4276 (87.63, 14.4272) -> (88.138, 14.4272)
  arc A2812 (87.884, 14.986) -> (87.884, 13.8684) centre (87.884, 14.4272) ccw
  arc A2813 (87.5538, 27.1272) -> (88.2142, 27.1272) centre (87.884, 27.1272) ccw
  line L4277 (87.63, 14.4272) -> (88.138, 14.4272)
  line L4278 (87.884, 14.1732) -> (87.884, 14.6812)
  arc A2814 (87.884, 14.986) -> (87.884, 13.8684) centre (87.884, 14.4272) ccw
  arc A2815 (87.884, 26.5684) -> (87.884, 27.686) centre (87.884, 27.1272) ccw
  arc A2816 (87.884, 26.5684) -> (87.884, 27.686) centre (87.884, 27.1272) ccw
  arc A2817 (88.2142, 14.4272) -> (87.5538, 14.4272) centre (87.884, 14.4272) ccw
  line L4279 (87.884, 14.1732) -> (87.884, 14.6812)
  line L4280 (87.884, 14.1732) -> (87.884, 14.6812)
  arc A2818 (87.5538, 14.4272) -> (88.2142, 14.4272) centre (87.884, 14.4272) ccw
  line L4281 (87.884, 14.1732) -> (87.884, 14.6812)
  line L4282 (87.884, 14.1732) -> (87.884, 14.6812)
  arc A2819 (87.884, 13.8684) -> (87.884, 14.986) centre (87.884, 14.4272) ccw
  line L4283 (87.63, 14.4272) -> (88.138, 14.4272)
  arc A2820 (87.884, 14.7765) -> (87.884, 14.0779) centre (87.884, 14.4272) ccw
  arc A2821 (87.884, 14.986) -> (87.884, 13.8684) centre (87.884, 14.4272) ccw
  arc A2822 (87.5538, 14.4272) -> (88.2142, 14.4272) centre (87.884, 14.4272) ccw
  line L4284 (87.884, 14.1732) -> (87.884, 14.6812)
  line L4285 (87.63, 14.4272) -> (88.138, 14.4272)
  arc A2823 (87.884, 13.8684) -> (87.884, 14.986) centre (87.884, 14.4272) ccw
  arc A2824 (87.884, 14.986) -> (87.884, 13.8684) centre (87.884, 14.4272) ccw
  arc A2825 (87.5538, 14.4272) -> (88.2142, 14.4272) centre (87.884, 14.4272) ccw
  arc A2826 (87.884, 26.5684) -> (87.884, 27.686) centre (87.884, 27.1272) ccw
  arc A2827 (87.5538, 14.4272) -> (88.2142, 14.4272) centre (87.884, 14.4272) ccw
  line L4286 (87.63, 14.4272) -> (88.138, 14.4272)
  arc A2828 (87.5538, 14.4272) -> (88.2142, 14.4272) centre (87.884, 14.4272) ccw
  arc A2829 (87.884, 14.0779) -> (87.884, 14.7765) centre (87.884, 14.4272) ccw
  line L4287 (87.884, 26.8732) -> (87.884, 27.3812)
  line L4288 (87.63, 27.1272) -> (88.138, 27.1272)
  line L4289 (87.63, 27.1272) -> (88.138, 27.1272)
  arc A2830 (88.2142, 27.1272) -> (87.5538, 27.1272) centre (87.884, 27.1272) ccw
  arc A2831 (87.884, 27.686) -> (87.884, 26.5684) centre (87.884, 27.1272) ccw
  arc A2832 (87.884, 14.986) -> (87.884, 13.8684) centre (87.884, 14.4272) ccw
  arc A2833 (88.2142, 14.4272) -> (87.5538, 14.4272) centre (87.884, 14.4272) ccw
  line L4290 (87.884, 26.8732) -> (87.884, 27.3812)
  line L4291 (87.63, 14.4272) -> (88.138, 14.4272)
  arc A2834 (86.7664, 14.4272) -> (89.0016, 14.4272) centre (87.884, 14.4272) ccw
  arc A2835 (88.2142, 14.4272) -> (87.5538, 14.4272) centre (87.884, 14.4272) ccw
  arc A2836 (88.2142, 14.4272) -> (87.5538, 14.4272) centre (87.884, 14.4272) ccw
  arc A2837 (87.884, 27.686) -> (87.884, 26.5684) centre (87.884, 27.1272) ccw
  arc A2838 (87.5538, 14.4272) -> (88.2142, 14.4272) centre (87.884, 14.4272) ccw
  arc A2839 (87.884, 13.8684) -> (87.884, 14.986) centre (87.884, 14.4272) ccw
  line L4292 (87.63, 14.4272) -> (88.138, 14.4272)
  line L4293 (87.63, 14.4272) -> (88.138, 14.4272)
  line L4294 (87.63, 14.4272) -> (88.138, 14.4272)
  arc A2840 (87.884, 13.8684) -> (87.884, 14.986) centre (87.884, 14.4272) ccw
  arc A2841 (87.5538, 14.4272) -> (88.2142, 14.4272) centre (87.884, 14.4272) ccw
  arc A2842 (88.2142, 14.4272) -> (87.5538, 14.4272) centre (87.884, 14.4272) ccw
  arc A2843 (88.2142, 14.4272) -> (87.5538, 14.4272) centre (87.884, 14.4272) ccw
  arc A2844 (88.2142, 14.4272) -> (87.5538, 14.4272) centre (87.884, 14.4272) ccw
  arc A2845 (86.7664, 14.4272) -> (89.0016, 14.4272) centre (87.884, 14.4272) ccw
  arc A2846 (87.5538, 14.4272) -> (88.2142, 14.4272) centre (87.884, 14.4272) ccw
  arc A2847 (57.5754, 11.5316) -> (57.0801, 11.5316) centre (57.3278, 11.5316) ccw
  line L4295 (55.4228, 13.0048) -> (55.4228, 10.0584)
  line L4296 (57.0738, 11.5316) -> (57.5818, 11.5316)
  arc A2848 (57.0801, 11.5316) -> (57.5754, 11.5316) centre (57.3278, 11.5316) ccw
  line L4297 (63.6778, 13.0048) -> (56.0578, 13.0048)
  line L4298 (40.8178, 61.341) -> (40.8178, 60.325)
  line L4299 (40.2082, 61.341) -> (40.8178, 61.341)
  line L4300 (64.3128, 10.0584) -> (64.3128, 13.0048)
  line L4301 (56.0578, 10.0584) -> (63.6778, 10.0584)
  arc A2849 (59.8678, 11.1379) -> (59.8678, 11.9253) centre (59.8678, 11.5316) ccw
  arc A2850 (60.1154, 11.5316) -> (59.6201, 11.5316) centre (59.8678, 11.5316) ccw
  line L4302 (40.2082, 60.325) -> (40.2082, 61.341)
  line L4303 (40.8178, 60.325) -> (40.2082, 60.325)
  arc A2851 (57.5754, 11.5316) -> (57.0801, 11.5316) centre (57.3278, 11.5316) ccw
  line L4304 (40.2082, 60.958) -> (40.2082, 60.708)
  line L4305 (57.0738, 11.5316) -> (57.5818, 11.5316)
  arc A2852 (57.0801, 11.5316) -> (57.5754, 11.5316) centre (57.3278, 11.5316) ccw
  arc A2853 (87.5538, 14.4272) -> (88.2142, 14.4272) centre (87.884, 14.4272) ccw
  arc A2854 (57.0801, 11.5316) -> (57.5754, 11.5316) centre (57.3278, 11.5316) ccw
  line L4306 (40.2082, 60.325) -> (40.2082, 61.341)
  line L4307 (63.6778, 10.0584) -> (63.6778, 13.0048)
  arc A2855 (57.0801, 11.5316) -> (57.5754, 11.5316) centre (57.3278, 11.5316) ccw
  arc A2856 (57.0801, 11.5316) -> (57.5754, 11.5316) centre (57.3278, 11.5316) ccw
  line L4308 (57.0738, 11.5316) -> (57.5818, 11.5316)
  line L4309 (40.2082, 61.341) -> (40.8178, 61.341)
  line L4310 (40.8178, 61.341) -> (40.8178, 60.325)
  line L4311 (57.0738, 11.5316) -> (57.5818, 11.5316)
  line L4312 (57.3278, 11.2776) -> (57.3278, 11.7856)
  arc A2857 (57.5754, 11.5316) -> (57.0801, 11.5316) centre (57.3278, 11.5316) ccw
  arc A2858 (57.0801, 11.5316) -> (57.5754, 11.5316) centre (57.3278, 11.5316) ccw
  line L4313 (87.884, 14.1732) -> (87.884, 14.6812)
  line L4314 (40.813, 60.283) -> (40.813, 61.383)
  line L4315 (57.3278, 11.2776) -> (57.3278, 11.7856)
  line L4316 (57.0738, 11.5316) -> (57.5818, 11.5316)
  arc A2859 (57.5754, 11.5316) -> (57.0801, 11.5316) centre (57.3278, 11.5316) ccw
  line L4317 (57.3278, 11.2776) -> (57.3278, 11.7856)
  line L4318 (40.213, 60.283) -> (40.813, 60.283)
  line L4319 (57.0738, 11.5316) -> (57.5818, 11.5316)
  arc A2860 (89.0016, 14.4272) -> (86.7664, 14.4272) centre (87.884, 14.4272) ccw
  line L4320 (40.8178, 60.958) -> (40.2082, 60.958)
  line L4321 (40.8178, 60.708) -> (40.8178, 60.958)
  line L4322 (40.813, 61.383) -> (40.213, 61.383)
  line L4323 (57.0738, 11.5316) -> (57.5818, 11.5316)
  line L4324 (40.2082, 60.708) -> (40.8178, 60.708)
  arc A2861 (87.884, 13.8684) -> (87.884, 14.986) centre (87.884, 14.4272) ccw
  line L4325 (57.3278, 11.2776) -> (57.3278, 11.7856)
  line L4326 (40.213, 61.383) -> (40.213, 60.283)
  arc A2862 (57.5754, 11.5316) -> (57.0801, 11.5316) centre (57.3278, 11.5316) ccw
  arc A2863 (57.0801, 11.5316) -> (57.5754, 11.5316) centre (57.3278, 11.5316) ccw
  line L4327 (64.3128, 13.0048) -> (55.4228, 13.0048)
  arc A2864 (57.5754, 11.5316) -> (57.0801, 11.5316) centre (57.3278, 11.5316) ccw
  line L4328 (56.0578, 13.0048) -> (56.0578, 10.0584)
  line L4329 (57.3278, 11.2776) -> (57.3278, 11.7856)
  arc A2865 (57.5754, 11.5316) -> (57.0801, 11.5316) centre (57.3278, 11.5316) ccw
  line L4330 (57.0738, 11.5316) -> (57.5818, 11.5316)
  line L4331 (57.3278, 11.2776) -> (57.3278, 11.7856)
  line L4332 (57.3278, 11.2776) -> (57.3278, 11.7856)
  line L4333 (40.8178, 60.325) -> (40.2082, 60.325)
  arc A2866 (57.0801, 11.5316) -> (57.5754, 11.5316) centre (57.3278, 11.5316) ccw
  arc A2867 (57.5754, 11.5316) -> (57.0801, 11.5316) centre (57.3278, 11.5316) ccw
  line L4334 (57.3278, 11.2776) -> (57.3278, 11.7856)
  line L4335 (55.4228, 10.0584) -> (64.3128, 10.0584)
  arc A2868 (57.0801, 11.5316) -> (57.5754, 11.5316) centre (57.3278, 11.5316) ccw
  arc A2869 (57.5754, 11.5316) -> (57.0801, 11.5316) centre (57.3278, 11.5316) ccw
  line L4336 (59.6138, 11.5316) -> (60.1218, 11.5316)
  line L4337 (59.8678, 11.2776) -> (59.8678, 11.7856)
  line L4338 (59.6138, 11.5316) -> (60.1218, 11.5316)
  line L4339 (59.6138, 11.5316) -> (60.1218, 11.5316)
  arc A2870 (57.3278, 11.7856) -> (57.3278, 11.2776) centre (57.3278, 11.5316) ccw
  arc A2871 (59.6201, 11.5316) -> (60.1154, 11.5316) centre (59.8678, 11.5316) ccw
  arc A2872 (59.6201, 11.5316) -> (60.1154, 11.5316) centre (59.8678, 11.5316) ccw
  line L4340 (59.6138, 11.5316) -> (60.1218, 11.5316)
  arc A2873 (62.1602, 11.5316) -> (62.6555, 11.5316) centre (62.4078, 11.5316) ccw
  line L4341 (62.1538, 11.5316) -> (62.6618, 11.5316)
  arc A2874 (62.1602, 11.5316) -> (62.6555, 11.5316) centre (62.4078, 11.5316) ccw
  arc A2875 (60.1154, 11.5316) -> (59.6201, 11.5316) centre (59.8678, 11.5316) ccw
  line L4342 (56.5404, 11.5316) -> (58.1152, 11.5316)
  arc A2876 (60.1154, 11.5316) -> (59.6201, 11.5316) centre (59.8678, 11.5316) ccw
  arc A2877 (60.1154, 11.5316) -> (59.6201, 11.5316) centre (59.8678, 11.5316) ccw
  arc A2878 (62.1602, 11.5316) -> (62.6555, 11.5316) centre (62.4078, 11.5316) ccw
  line L4343 (59.8678, 11.2776) -> (59.8678, 11.7856)
  line L4344 (59.8678, 11.2776) -> (59.8678, 11.7856)
  arc A2879 (59.6201, 11.5316) -> (60.1154, 11.5316) centre (59.8678, 11.5316) ccw
  line L4345 (57.0738, 11.5316) -> (57.5818, 11.5316)
  arc A2880 (59.8678, 11.1379) -> (59.8678, 11.9253) centre (59.8678, 11.5316) ccw
  line L4346 (59.8678, 11.2776) -> (59.8678, 11.7856)
  arc A2881 (62.1602, 11.5316) -> (62.6555, 11.5316) centre (62.4078, 11.5316) ccw
  arc A2882 (62.4078, 11.9253) -> (62.4078, 11.1379) centre (62.4078, 11.5316) ccw
  arc A2883 (62.6555, 11.5316) -> (62.1602, 11.5316) centre (62.4078, 11.5316) ccw
  arc A2884 (62.4078, 11.1379) -> (62.4078, 11.9253) centre (62.4078, 11.5316) ccw
  arc A2885 (60.1154, 11.5316) -> (59.6201, 11.5316) centre (59.8678, 11.5316) ccw
  arc A2886 (59.8678, 11.1379) -> (59.8678, 11.9253) centre (59.8678, 11.5316) ccw
  line L4347 (59.6138, 11.5316) -> (60.1218, 11.5316)
  arc A2887 (59.6201, 11.5316) -> (60.1154, 11.5316) centre (59.8678, 11.5316) ccw
  arc A2888 (60.1154, 11.5316) -> (59.6201, 11.5316) centre (59.8678, 11.5316) ccw
  line L4348 (59.6138, 11.5316) -> (60.1218, 11.5316)
  line L4349 (59.6138, 11.5316) -> (60.1218, 11.5316)
  arc A2889 (59.6201, 11.5316) -> (60.1154, 11.5316) centre (59.8678, 11.5316) ccw
  arc A2890 (60.1154, 11.5316) -> (59.6201, 11.5316) centre (59.8678, 11.5316) ccw
  line L4350 (59.8678, 11.2776) -> (59.8678, 11.7856)
  arc A2891 (60.1154, 11.5316) -> (59.6201, 11.5316) centre (59.8678, 11.5316) ccw
  line L4351 (59.6138, 11.5316) -> (60.1218, 11.5316)
  arc A2892 (57.3278, 11.2776) -> (57.3278, 11.7856) centre (57.3278, 11.5316) ccw
  arc A2893 (60.1154, 11.5316) -> (59.6201, 11.5316) centre (59.8678, 11.5316) ccw
  line L4352 (59.8678, 11.2776) -> (59.8678, 11.7856)
  line L4353 (59.8678, 11.2776) -> (59.8678, 11.7856)
  line L4354 (59.8678, 11.2776) -> (59.8678, 11.7856)
  arc A2894 (60.1154, 11.5316) -> (59.6201, 11.5316) centre (59.8678, 11.5316) ccw
  arc A2895 (57.3278, 11.1379) -> (57.3278, 11.9253) centre (57.3278, 11.5316) ccw
  arc A2896 (59.6201, 11.5316) -> (60.1154, 11.5316) centre (59.8678, 11.5316) ccw
  line L4355 (56.5404, 11.5316) -> (58.1152, 11.5316)
  line L4356 (59.6138, 11.5316) -> (60.1218, 11.5316)
  line L4357 (59.8678, 11.2776) -> (59.8678, 11.7856)
  arc A2897 (57.0801, 11.5316) -> (57.5754, 11.5316) centre (57.3278, 11.5316) ccw
  arc A2898 (59.8678, 11.9253) -> (59.8678, 11.1379) centre (59.8678, 11.5316) ccw
  arc A2899 (59.6201, 11.5316) -> (60.1154, 11.5316) centre (59.8678, 11.5316) ccw
  line L4358 (57.3278, 11.2776) -> (57.3278, 11.7856)
  line L4359 (56.5404, 11.5316) -> (58.1152, 11.5316)
  arc A2900 (57.5754, 11.5316) -> (57.0801, 11.5316) centre (57.3278, 11.5316) ccw
  arc A2901 (59.6201, 11.5316) -> (60.1154, 11.5316) centre (59.8678, 11.5316) ccw
  arc A2902 (59.6201, 11.5316) -> (60.1154, 11.5316) centre (59.8678, 11.5316) ccw
  arc A2903 (59.6201, 11.5316) -> (60.1154, 11.5316) centre (59.8678, 11.5316) ccw
  arc A2904 (57.3278, 11.9253) -> (57.3278, 11.1379) centre (57.3278, 11.5316) ccw
  line L4360 (57.0738, 11.5316) -> (57.5818, 11.5316)
  line L4361 (59.6138, 11.5316) -> (60.1218, 11.5316)
  line L4362 (57.3278, 11.2776) -> (57.3278, 11.7856)
  line L4363 (56.5404, 11.5316) -> (58.1152, 11.5316)
  line L4364 (59.8678, 11.2776) -> (59.8678, 11.7856)
  line L4365 (41.36, 60.498) -> (41.36, 59.898)
  line L4366 (48.9686, 60.8698) -> (48.0086, 60.8698)
  arc A2905 (59.8678, 11.9253) -> (59.8678, 11.1379) centre (59.8678, 11.5316) ccw
  arc A2906 (59.8678, 11.1379) -> (59.8678, 11.9253) centre (59.8678, 11.5316) ccw
  arc A2907 (62.4078, 11.9253) -> (62.4078, 11.1379) centre (62.4078, 11.5316) ccw
  line L4367 (62.1538, 11.5316) -> (62.6618, 11.5316)
  line L4368 (62.1538, 11.5316) -> (62.6618, 11.5316)
  arc A2908 (62.6555, 11.5316) -> (62.1602, 11.5316) centre (62.4078, 11.5316) ccw
  arc A2909 (48.26, 58.1104) -> (48.26, 58.0088) centre (48.26, 58.0596) ccw
  line L4369 (48.9386, 59.2948) -> (48.0386, 59.2948)
  line L4370 (48.1886, 56.1428) -> (48.7886, 56.1428)
  line L4371 (48.7934, 56.5678) -> (48.7934, 56.8178)
  arc A2910 (59.8678, 11.9253) -> (59.8678, 11.1379) centre (59.8678, 11.5316) ccw
  line L4372 (48.0086, 60.8698) -> (48.0086, 59.1198)
  line L4373 (41.36, 59.898) -> (42.46, 59.898)
  line L4374 (48.006, 60.833) -> (48.006, 59.1566)
  arc A2911 (62.4078, 11.2776) -> (62.4078, 11.7856) centre (62.4078, 11.5316) ccw
  line L4375 (48.0086, 59.1198) -> (48.9686, 59.1198)
  arc A2912 (59.8678, 11.1379) -> (59.8678, 11.9253) centre (59.8678, 11.5316) ccw
  line L4376 (62.4078, 11.2776) -> (62.4078, 11.7856)
  line L4377 (48.1838, 56.8178) -> (48.1838, 56.5678)
  line L4378 (42.418, 60.5028) -> (42.418, 59.8932)
  line L4379 (48.9386, 60.6948) -> (48.0386, 60.6948)
  line L4380 (42.46, 60.498) -> (41.36, 60.498)
  line L4381 (48.1838, 57.2008) -> (48.7934, 57.2008)
  arc A2913 (48.26, 58.0088) -> (48.26, 58.1104) centre (48.26, 58.0596) ccw
  line L4382 (48.9386, 59.2948) -> (48.0386, 59.2948)
  line L4383 (48.1838, 56.5678) -> (48.7934, 56.5678)
  arc A2914 (62.4078, 11.7856) -> (62.4078, 11.2776) centre (62.4078, 11.5316) ccw
  arc A2915 (62.4078, 11.1379) -> (62.4078, 11.9253) centre (62.4078, 11.5316) ccw
  arc A2916 (62.4078, 11.1379) -> (62.4078, 11.9253) centre (62.4078, 11.5316) ccw
  line L4384 (48.9686, 59.1198) -> (48.9686, 60.8698)
  arc A2917 (62.6555, 11.5316) -> (62.1602, 11.5316) centre (62.4078, 11.5316) ccw
  line L4385 (62.4078, 11.2776) -> (62.4078, 11.7856)
  arc A2918 (59.8678, 11.9253) -> (59.8678, 11.1379) centre (59.8678, 11.5316) ccw
  line L4386 (62.1538, 11.5316) -> (62.6618, 11.5316)
  line L4387 (48.006, 60.833) -> (48.006, 59.1566)
  arc A2919 (62.6555, 11.5316) -> (62.1602, 11.5316) centre (62.4078, 11.5316) ccw
  arc A2920 (62.4078, 11.1379) -> (62.4078, 11.9253) centre (62.4078, 11.5316) ccw
  line L4388 (48.006, 59.1566) -> (48.9712, 59.1566)
  arc A2921 (62.6555, 11.5316) -> (62.1602, 11.5316) centre (62.4078, 11.5316) ccw
  line L4389 (62.4078, 11.2776) -> (62.4078, 11.7856)